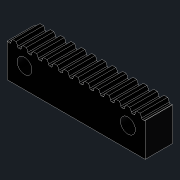
# Autodesk Inventor part: base37
Saved by Autodesk Inventor 2022 (Build 260153000, 153)
## iProperties
Created: 2021-08-06
Part Number: base37
Material: ABS プラスチック
Document SubType Name: Modeling
Designer: yuta0
Density: 1.06 g/cm^3
Appearance: 滑らか - 黒
Mass: 7.28168 g
Surface Area: 31.8793 cm^2
Volume: 6.86951 cm^3
購入先: 印刷
在庫数: 0.0
Author: yuta0
Autodesk Inventor part; units mm, degrees
(part 1 of 2)
ref_plane "YZ Plane" through (0, 0, 0) normal (1, 0, 0) x (0, 1, 0)
ref_plane "XZ Plane" through (0, 0, 0) normal (0, 1, 0) x (-1, 0, 0)
ref_plane "XY Plane" through (0, 0, 0) normal (0, 0, 1) x (1, 0, 0)
sketch "スケッチ1" plane through (0, 0, 0) normal (0, 0, 1) x (1, 0, 0)
  line L0 (-20, -5) -> (20, -5)
  line L1 (20, -5) -> (20, 9)
  line L2 (20, 9) -> (-20, 9)
  line L3 (-20, 9) -> (-20, -5)
  point P0 (0, 0)
  dimension "d0" = 40
  dimension "d66" = 5
  dimension "d67" = 9
  dimension "d68" = 20
  constraints: 8 end point, 2 parallel, 1 horizontal, 1 perpendicular
  measures "d0" distance of L0.start L0.end
  measures "d66" distance from line of L0 point (0, 0)
  measures "d67" distance from line of L2 point (0, 0)
  measures "d68" distance from line of L1 point (0, 0)
extrude "押し出し1" add sketch "スケッチ1" along normal blind 8
sketch "スケッチ2" plane through (0, 0, 8) normal (0, 0, 1) x (1, 0, 0)
  line L0 (-50, -10) -> (50, -10) construction
  line L1 (-50, -26.2338) -> (50, -26.2338) construction
  line L2 (50, 6.2338) -> (-50, 6.2338) construction
  arc A0 (-50, 6.2338) -> (-50, -26.2338) centre (-50, -10) ccw construction
  arc A1 (50, -26.2338) -> (50, 6.2338) centre (50, -10) ccw construction
  line L3 (-50, 6.6528) -> (50, 6.6528)
  arc A2 (50, -26.6528) -> (50, 6.6528) centre (50, -10) ccw
  line L4 (50, -26.6528) -> (-50, -26.6528)
  arc A3 (-50, 6.6528) -> (-50, -26.6528) centre (-50, -10) ccw
  line L5 (-50, -25.8528) -> (50, -25.8528)
  arc A4 (50, -25.8528) -> (50, 5.8528) centre (50, -10) ccw
  line L6 (50, 5.8528) -> (-50, 5.8528) construction
  arc A5 (-50, 5.8528) -> (-50, -25.8528) centre (-50, -10) ccw
  line L7 (-1.5, 4.6028) -> (-1.2549, 4.6028)
  arc A6 (-1.2549, 4.6028) -> (-0.9576, 4.8628) centre (-1.2549, 4.9028) ccw
  arc A7 (-0.5217, 5.8528) -> (-0.9576, 4.8628) centre (0.975, 4.6028) ccw
  line L8 (-0.5217, 5.8528) -> (0.5217, 5.8528)
  arc A8 (0.9576, 4.8628) -> (0.5217, 5.8528) centre (-0.975, 4.6028) ccw
  arc A9 (0.9576, 4.8628) -> (1.2549, 4.6028) centre (1.2549, 4.9028) ccw
  line L9 (1.2549, 4.6028) -> (1.5, 4.6028)
  line L10 (-20, 9) -> (-20, -5) projected
  line L11 (20, 9) -> (-20, 9) projected
  line L12 (20, -5) -> (20, 9) projected
  arc A10 (-2.0424, 4.8628) -> (-1.7451, 4.6028) centre (-1.7451, 4.9028) ccw
  arc A11 (-4.2549, 4.6028) -> (-3.9576, 4.8628) centre (-4.2549, 4.9028) ccw
  line L13 (-4.5, 4.6028) -> (-4.2549, 4.6028)
  line L14 (-1.7451, 4.6028) -> (-1.5, 4.6028)
  arc A12 (-2.0424, 4.8628) -> (-2.4783, 5.8528) centre (-3.975, 4.6028) ccw
  line L15 (-3.5217, 5.8528) -> (-2.4783, 5.8528)
  arc A13 (-3.5217, 5.8528) -> (-3.9576, 4.8628) centre (-2.025, 4.6028) ccw
  arc A14 (-5.0424, 4.8628) -> (-4.7451, 4.6028) centre (-4.7451, 4.9028) ccw
  arc A15 (-7.2549, 4.6028) -> (-6.9576, 4.8628) centre (-7.2549, 4.9028) ccw
  line L16 (-7.5, 4.6028) -> (-7.2549, 4.6028)
  line L17 (-4.7451, 4.6028) -> (-4.5, 4.6028)
  arc A16 (-5.0424, 4.8628) -> (-5.4783, 5.8528) centre (-6.975, 4.6028) ccw
  line L18 (-6.5217, 5.8528) -> (-5.4783, 5.8528)
  arc A17 (-6.5217, 5.8528) -> (-6.9576, 4.8628) centre (-5.025, 4.6028) ccw
  arc A18 (-8.0424, 4.8628) -> (-7.7451, 4.6028) centre (-7.7451, 4.9028) ccw
  arc A19 (-10.2549, 4.6028) -> (-9.9576, 4.8628) centre (-10.2549, 4.9028) ccw
  line L19 (-10.5, 4.6028) -> (-10.2549, 4.6028)
  line L20 (-7.7451, 4.6028) -> (-7.5, 4.6028)
  arc A20 (-8.0424, 4.8628) -> (-8.4783, 5.8528) centre (-9.975, 4.6028) ccw
  line L21 (-9.5217, 5.8528) -> (-8.4783, 5.8528)
  arc A21 (-9.5217, 5.8528) -> (-9.9576, 4.8628) centre (-8.025, 4.6028) ccw
  arc A22 (-11.0424, 4.8628) -> (-10.7451, 4.6028) centre (-10.7451, 4.9028) ccw
  arc A23 (-13.2549, 4.6028) -> (-12.9576, 4.8628) centre (-13.2549, 4.9028) ccw
  line L22 (-13.5, 4.6028) -> (-13.2549, 4.6028)
  line L23 (-10.7451, 4.6028) -> (-10.5, 4.6028)
  arc A24 (-11.0424, 4.8628) -> (-11.4783, 5.8528) centre (-12.975, 4.6028) ccw
  line L24 (-12.5217, 5.8528) -> (-11.4783, 5.8528)
  arc A25 (-12.5217, 5.8528) -> (-12.9576, 4.8628) centre (-11.025, 4.6028) ccw
  arc A26 (-14.0424, 4.8628) -> (-13.7451, 4.6028) centre (-13.7451, 4.9028) ccw
  arc A27 (-16.2549, 4.6028) -> (-15.9576, 4.8628) centre (-16.2549, 4.9028) ccw
  line L25 (-16.5, 4.6028) -> (-16.2549, 4.6028)
  line L26 (-13.7451, 4.6028) -> (-13.5, 4.6028)
  arc A28 (-14.0424, 4.8628) -> (-14.4783, 5.8528) centre (-15.975, 4.6028) ccw
  line L27 (-15.5217, 5.8528) -> (-14.4783, 5.8528)
  arc A29 (-15.5217, 5.8528) -> (-15.9576, 4.8628) centre (-14.025, 4.6028) ccw
  arc A30 (-17.0424, 4.8628) -> (-16.7451, 4.6028) centre (-16.7451, 4.9028) ccw
  arc A31 (-19.2549, 4.6028) -> (-18.9576, 4.8628) centre (-19.2549, 4.9028) ccw
  line L28 (-19.5, 4.6028) -> (-19.2549, 4.6028)
  line L29 (-16.7451, 4.6028) -> (-16.5, 4.6028)
  arc A32 (-17.0424, 4.8628) -> (-17.4783, 5.8528) centre (-18.975, 4.6028) ccw
  line L30 (-18.5217, 5.8528) -> (-17.4783, 5.8528)
  arc A33 (-18.5217, 5.8528) -> (-18.9576, 4.8628) centre (-17.025, 4.6028) ccw
  arc A34 (-20.0424, 4.8628) -> (-19.7451, 4.6028) centre (-19.7451, 4.9028) ccw
  arc A35 (-22.2549, 4.6028) -> (-21.9576, 4.8628) centre (-22.2549, 4.9028) ccw
  line L31 (-22.5, 4.6028) -> (-22.2549, 4.6028)
  line L32 (-19.7451, 4.6028) -> (-19.5, 4.6028)
  arc A36 (-20.0424, 4.8628) -> (-20.4783, 5.8528) centre (-21.975, 4.6028) ccw
  line L33 (-21.5217, 5.8528) -> (-20.4783, 5.8528)
  arc A37 (-21.5217, 5.8528) -> (-21.9576, 4.8628) centre (-20.025, 4.6028) ccw
  arc A38 (-23.0424, 4.8628) -> (-22.7451, 4.6028) centre (-22.7451, 4.9028) ccw
  arc A39 (-25.2549, 4.6028) -> (-24.9576, 4.8628) centre (-25.2549, 4.9028) ccw
  line L34 (-25.5, 4.6028) -> (-25.2549, 4.6028)
  line L35 (-22.7451, 4.6028) -> (-22.5, 4.6028)
  arc A40 (-23.0424, 4.8628) -> (-23.4783, 5.8528) centre (-24.975, 4.6028) ccw
  line L36 (-24.5217, 5.8528) -> (-23.4783, 5.8528)
  arc A41 (-24.5217, 5.8528) -> (-24.9576, 4.8628) centre (-23.025, 4.6028) ccw
  arc A42 (-26.0424, 4.8628) -> (-25.7451, 4.6028) centre (-25.7451, 4.9028) ccw
  arc A43 (-28.2549, 4.6028) -> (-27.9576, 4.8628) centre (-28.2549, 4.9028) ccw
  line L37 (-28.5, 4.6028) -> (-28.2549, 4.6028)
  line L38 (-25.7451, 4.6028) -> (-25.5, 4.6028)
  arc A44 (-26.0424, 4.8628) -> (-26.4783, 5.8528) centre (-27.975, 4.6028) ccw
  line L39 (-27.5217, 5.8528) -> (-26.4783, 5.8528)
  arc A45 (-27.5217, 5.8528) -> (-27.9576, 4.8628) centre (-26.025, 4.6028) ccw
  arc A46 (3.9576, 4.8628) -> (4.2549, 4.6028) centre (4.2549, 4.9028) ccw
  arc A47 (1.7451, 4.6028) -> (2.0424, 4.8628) centre (1.7451, 4.9028) ccw
  line L40 (1.5, 4.6028) -> (1.7451, 4.6028)
  line L41 (4.2549, 4.6028) -> (4.5, 4.6028)
  arc A48 (3.9576, 4.8628) -> (3.5217, 5.8528) centre (2.025, 4.6028) ccw
  line L42 (2.4783, 5.8528) -> (3.5217, 5.8528)
  arc A49 (2.4783, 5.8528) -> (2.0424, 4.8628) centre (3.975, 4.6028) ccw
  arc A50 (0.9576, 4.8628) -> (1.2549, 4.6028) centre (1.2549, 4.9028) ccw
  arc A51 (-1.2549, 4.6028) -> (-0.9576, 4.8628) centre (-1.2549, 4.9028) ccw
  line L43 (-1.5, 4.6028) -> (-1.2549, 4.6028)
  line L44 (1.2549, 4.6028) -> (1.5, 4.6028)
  arc A52 (0.9576, 4.8628) -> (0.5217, 5.8528) centre (-0.975, 4.6028) ccw
  line L45 (-0.5217, 5.8528) -> (0.5217, 5.8528)
  arc A53 (-0.5217, 5.8528) -> (-0.9576, 4.8628) centre (0.975, 4.6028) ccw
  arc A54 (-2.0424, 4.8628) -> (-1.7451, 4.6028) centre (-1.7451, 4.9028) ccw
  arc A55 (-4.2549, 4.6028) -> (-3.9576, 4.8628) centre (-4.2549, 4.9028) ccw
  line L46 (-4.5, 4.6028) -> (-4.2549, 4.6028)
  line L47 (-1.7451, 4.6028) -> (-1.5, 4.6028)
  arc A56 (-2.0424, 4.8628) -> (-2.4783, 5.8528) centre (-3.975, 4.6028) ccw
  line L48 (-3.5217, 5.8528) -> (-2.4783, 5.8528)
  arc A57 (-3.5217, 5.8528) -> (-3.9576, 4.8628) centre (-2.025, 4.6028) ccw
  arc A58 (-5.0424, 4.8628) -> (-4.7451, 4.6028) centre (-4.7451, 4.9028) ccw
  arc A59 (-7.2549, 4.6028) -> (-6.9576, 4.8628) centre (-7.2549, 4.9028) ccw
  line L49 (-7.5, 4.6028) -> (-7.2549, 4.6028)
  line L50 (-4.7451, 4.6028) -> (-4.5, 4.6028)
  arc A60 (-5.0424, 4.8628) -> (-5.4783, 5.8528) centre (-6.975, 4.6028) ccw
  line L51 (-6.5217, 5.8528) -> (-5.4783, 5.8528)
  arc A61 (-6.5217, 5.8528) -> (-6.9576, 4.8628) centre (-5.025, 4.6028) ccw
  arc A62 (-8.0424, 4.8628) -> (-7.7451, 4.6028) centre (-7.7451, 4.9028) ccw
  arc A63 (-10.2549, 4.6028) -> (-9.9576, 4.8628) centre (-10.2549, 4.9028) ccw
  line L52 (-10.5, 4.6028) -> (-10.2549, 4.6028)
  line L53 (-7.7451, 4.6028) -> (-7.5, 4.6028)
  arc A64 (-8.0424, 4.8628) -> (-8.4783, 5.8528) centre (-9.975, 4.6028) ccw
  line L54 (-9.5217, 5.8528) -> (-8.4783, 5.8528)
  arc A65 (-9.5217, 5.8528) -> (-9.9576, 4.8628) centre (-8.025, 4.6028) ccw
  arc A66 (-11.0424, 4.8628) -> (-10.7451, 4.6028) centre (-10.7451, 4.9028) ccw
  arc A67 (-13.2549, 4.6028) -> (-12.9576, 4.8628) centre (-13.2549, 4.9028) ccw
  line L55 (-13.5, 4.6028) -> (-13.2549, 4.6028)
  line L56 (-10.7451, 4.6028) -> (-10.5, 4.6028)
  arc A68 (-11.0424, 4.8628) -> (-11.4783, 5.8528) centre (-12.975, 4.6028) ccw
  line L57 (-12.5217, 5.8528) -> (-11.4783, 5.8528)
  arc A69 (-12.5217, 5.8528) -> (-12.9576, 4.8628) centre (-11.025, 4.6028) ccw
  arc A70 (-14.0424, 4.8628) -> (-13.7451, 4.6028) centre (-13.7451, 4.9028) ccw
  arc A71 (-16.2549, 4.6028) -> (-15.9576, 4.8628) centre (-16.2549, 4.9028) ccw
  line L58 (-16.5, 4.6028) -> (-16.2549, 4.6028)
  line L59 (-13.7451, 4.6028) -> (-13.5, 4.6028)
  arc A72 (-14.0424, 4.8628) -> (-14.4783, 5.8528) centre (-15.975, 4.6028) ccw
  line L60 (-15.5217, 5.8528) -> (-14.4783, 5.8528)
  arc A73 (-15.5217, 5.8528) -> (-15.9576, 4.8628) centre (-14.025, 4.6028) ccw
  arc A74 (-17.0424, 4.8628) -> (-16.7451, 4.6028) centre (-16.7451, 4.9028) ccw
  arc A75 (-19.2549, 4.6028) -> (-18.9576, 4.8628) centre (-19.2549, 4.9028) ccw
  line L61 (-19.5, 4.6028) -> (-19.2549, 4.6028)
  line L62 (-16.7451, 4.6028) -> (-16.5, 4.6028)
  arc A76 (-17.0424, 4.8628) -> (-17.4783, 5.8528) centre (-18.975, 4.6028) ccw
  line L63 (-18.5217, 5.8528) -> (-17.4783, 5.8528)
  arc A77 (-18.5217, 5.8528) -> (-18.9576, 4.8628) centre (-17.025, 4.6028) ccw
  arc A78 (-20.0424, 4.8628) -> (-19.7451, 4.6028) centre (-19.7451, 4.9028) ccw
  arc A79 (-22.2549, 4.6028) -> (-21.9576, 4.8628) centre (-22.2549, 4.9028) ccw
  line L64 (-22.5, 4.6028) -> (-22.2549, 4.6028)
  line L65 (-19.7451, 4.6028) -> (-19.5, 4.6028)
  arc A80 (-20.0424, 4.8628) -> (-20.4783, 5.8528) centre (-21.975, 4.6028) ccw
  line L66 (-21.5217, 5.8528) -> (-20.4783, 5.8528)
  arc A81 (-21.5217, 5.8528) -> (-21.9576, 4.8628) centre (-20.025, 4.6028) ccw
  arc A82 (-23.0424, 4.8628) -> (-22.7451, 4.6028) centre (-22.7451, 4.9028) ccw
  arc A83 (-25.2549, 4.6028) -> (-24.9576, 4.8628) centre (-25.2549, 4.9028) ccw
  line L67 (-25.5, 4.6028) -> (-25.2549, 4.6028)
  line L68 (-22.7451, 4.6028) -> (-22.5, 4.6028)
  arc A84 (-23.0424, 4.8628) -> (-23.4783, 5.8528) centre (-24.975, 4.6028) ccw
  line L69 (-24.5217, 5.8528) -> (-23.4783, 5.8528)
  arc A85 (-24.5217, 5.8528) -> (-24.9576, 4.8628) centre (-23.025, 4.6028) ccw
  arc A86 (6.9576, 4.8628) -> (7.2549, 4.6028) centre (7.2549, 4.9028) ccw
  arc A87 (4.7451, 4.6028) -> (5.0424, 4.8628) centre (4.7451, 4.9028) ccw
  line L70 (4.5, 4.6028) -> (4.7451, 4.6028)
  line L71 (7.2549, 4.6028) -> (7.5, 4.6028)
  arc A88 (6.9576, 4.8628) -> (6.5217, 5.8528) centre (5.025, 4.6028) ccw
  line L72 (5.4783, 5.8528) -> (6.5217, 5.8528)
  arc A89 (5.4783, 5.8528) -> (5.0424, 4.8628) centre (6.975, 4.6028) ccw
  arc A90 (3.9576, 4.8628) -> (4.2549, 4.6028) centre (4.2549, 4.9028) ccw
  arc A91 (1.7451, 4.6028) -> (2.0424, 4.8628) centre (1.7451, 4.9028) ccw
  line L73 (1.5, 4.6028) -> (1.7451, 4.6028)
  line L74 (4.2549, 4.6028) -> (4.5, 4.6028)
  arc A92 (3.9576, 4.8628) -> (3.5217, 5.8528) centre (2.025, 4.6028) ccw
  line L75 (2.4783, 5.8528) -> (3.5217, 5.8528)
  arc A93 (2.4783, 5.8528) -> (2.0424, 4.8628) centre (3.975, 4.6028) ccw
  arc A94 (0.9576, 4.8628) -> (1.2549, 4.6028) centre (1.2549, 4.9028) ccw
  arc A95 (-1.2549, 4.6028) -> (-0.9576, 4.8628) centre (-1.2549, 4.9028) ccw
  line L76 (-1.5, 4.6028) -> (-1.2549, 4.6028)
  line L77 (1.2549, 4.6028) -> (1.5, 4.6028)
  arc A96 (0.9576, 4.8628) -> (0.5217, 5.8528) centre (-0.975, 4.6028) ccw
  line L78 (-0.5217, 5.8528) -> (0.5217, 5.8528)
  arc A97 (-0.5217, 5.8528) -> (-0.9576, 4.8628) centre (0.975, 4.6028) ccw
  arc A98 (-2.0424, 4.8628) -> (-1.7451, 4.6028) centre (-1.7451, 4.9028) ccw
  arc A99 (-4.2549, 4.6028) -> (-3.9576, 4.8628) centre (-4.2549, 4.9028) ccw
  line L79 (-4.5, 4.6028) -> (-4.2549, 4.6028)
  line L80 (-1.7451, 4.6028) -> (-1.5, 4.6028)
  arc A100 (-2.0424, 4.8628) -> (-2.4783, 5.8528) centre (-3.975, 4.6028) ccw
  line L81 (-3.5217, 5.8528) -> (-2.4783, 5.8528)
  arc A101 (-3.5217, 5.8528) -> (-3.9576, 4.8628) centre (-2.025, 4.6028) ccw
  arc A102 (-5.0424, 4.8628) -> (-4.7451, 4.6028) centre (-4.7451, 4.9028) ccw
  arc A103 (-7.2549, 4.6028) -> (-6.9576, 4.8628) centre (-7.2549, 4.9028) ccw
  line L82 (-7.5, 4.6028) -> (-7.2549, 4.6028)
  line L83 (-4.7451, 4.6028) -> (-4.5, 4.6028)
  arc A104 (-5.0424, 4.8628) -> (-5.4783, 5.8528) centre (-6.975, 4.6028) ccw
  line L84 (-6.5217, 5.8528) -> (-5.4783, 5.8528)
  arc A105 (-6.5217, 5.8528) -> (-6.9576, 4.8628) centre (-5.025, 4.6028) ccw
  arc A106 (-8.0424, 4.8628) -> (-7.7451, 4.6028) centre (-7.7451, 4.9028) ccw
  arc A107 (-10.2549, 4.6028) -> (-9.9576, 4.8628) centre (-10.2549, 4.9028) ccw
  line L85 (-10.5, 4.6028) -> (-10.2549, 4.6028)
  line L86 (-7.7451, 4.6028) -> (-7.5, 4.6028)
  arc A108 (-8.0424, 4.8628) -> (-8.4783, 5.8528) centre (-9.975, 4.6028) ccw
  line L87 (-9.5217, 5.8528) -> (-8.4783, 5.8528)
  arc A109 (-9.5217, 5.8528) -> (-9.9576, 4.8628) centre (-8.025, 4.6028) ccw
  arc A110 (-11.0424, 4.8628) -> (-10.7451, 4.6028) centre (-10.7451, 4.9028) ccw
  arc A111 (-13.2549, 4.6028) -> (-12.9576, 4.8628) centre (-13.2549, 4.9028) ccw
  line L88 (-13.5, 4.6028) -> (-13.2549, 4.6028)
  line L89 (-10.7451, 4.6028) -> (-10.5, 4.6028)
  arc A112 (-11.0424, 4.8628) -> (-11.4783, 5.8528) centre (-12.975, 4.6028) ccw
  line L90 (-12.5217, 5.8528) -> (-11.4783, 5.8528)
  arc A113 (-12.5217, 5.8528) -> (-12.9576, 4.8628) centre (-11.025, 4.6028) ccw
  arc A114 (-14.0424, 4.8628) -> (-13.7451, 4.6028) centre (-13.7451, 4.9028) ccw
  arc A115 (-16.2549, 4.6028) -> (-15.9576, 4.8628) centre (-16.2549, 4.9028) ccw
  line L91 (-16.5, 4.6028) -> (-16.2549, 4.6028)
  line L92 (-13.7451, 4.6028) -> (-13.5, 4.6028)
  arc A116 (-14.0424, 4.8628) -> (-14.4783, 5.8528) centre (-15.975, 4.6028) ccw
  line L93 (-15.5217, 5.8528) -> (-14.4783, 5.8528)
  arc A117 (-15.5217, 5.8528) -> (-15.9576, 4.8628) centre (-14.025, 4.6028) ccw
  arc A118 (-17.0424, 4.8628) -> (-16.7451, 4.6028) centre (-16.7451, 4.9028) ccw
  arc A119 (-19.2549, 4.6028) -> (-18.9576, 4.8628) centre (-19.2549, 4.9028) ccw
  line L94 (-19.5, 4.6028) -> (-19.2549, 4.6028)
  line L95 (-16.7451, 4.6028) -> (-16.5, 4.6028)
  arc A120 (-17.0424, 4.8628) -> (-17.4783, 5.8528) centre (-18.975, 4.6028) ccw
  line L96 (-18.5217, 5.8528) -> (-17.4783, 5.8528)
  arc A121 (-18.5217, 5.8528) -> (-18.9576, 4.8628) centre (-17.025, 4.6028) ccw
  arc A122 (-20.0424, 4.8628) -> (-19.7451, 4.6028) centre (-19.7451, 4.9028) ccw
  arc A123 (-22.2549, 4.6028) -> (-21.9576, 4.8628) centre (-22.2549, 4.9028) ccw
  line L97 (-22.5, 4.6028) -> (-22.2549, 4.6028)
  line L98 (-19.7451, 4.6028) -> (-19.5, 4.6028)
  arc A124 (-20.0424, 4.8628) -> (-20.4783, 5.8528) centre (-21.975, 4.6028) ccw
  line L99 (-21.5217, 5.8528) -> (-20.4783, 5.8528)
  arc A125 (-21.5217, 5.8528) -> (-21.9576, 4.8628) centre (-20.025, 4.6028) ccw
  arc A126 (9.9576, 4.8628) -> (10.2549, 4.6028) centre (10.2549, 4.9028) ccw
  arc A127 (7.7451, 4.6028) -> (8.0424, 4.8628) centre (7.7451, 4.9028) ccw
  line L100 (7.5, 4.6028) -> (7.7451, 4.6028)
  line L101 (10.2549, 4.6028) -> (10.5, 4.6028)
  arc A128 (9.9576, 4.8628) -> (9.5217, 5.8528) centre (8.025, 4.6028) ccw
  line L102 (8.4783, 5.8528) -> (9.5217, 5.8528)
  arc A129 (8.4783, 5.8528) -> (8.0424, 4.8628) centre (9.975, 4.6028) ccw
  arc A130 (6.9576, 4.8628) -> (7.2549, 4.6028) centre (7.2549, 4.9028) ccw
  arc A131 (4.7451, 4.6028) -> (5.0424, 4.8628) centre (4.7451, 4.9028) ccw
  line L103 (4.5, 4.6028) -> (4.7451, 4.6028)
  line L104 (7.2549, 4.6028) -> (7.5, 4.6028)
  arc A132 (6.9576, 4.8628) -> (6.5217, 5.8528) centre (5.025, 4.6028) ccw
  line L105 (5.4783, 5.8528) -> (6.5217, 5.8528)
  arc A133 (5.4783, 5.8528) -> (5.0424, 4.8628) centre (6.975, 4.6028) ccw
  arc A134 (3.9576, 4.8628) -> (4.2549, 4.6028) centre (4.2549, 4.9028) ccw
  arc A135 (1.7451, 4.6028) -> (2.0424, 4.8628) centre (1.7451, 4.9028) ccw
  line L106 (1.5, 4.6028) -> (1.7451, 4.6028)
  line L107 (4.2549, 4.6028) -> (4.5, 4.6028)
  arc A136 (3.9576, 4.8628) -> (3.5217, 5.8528) centre (2.025, 4.6028) ccw
  line L108 (2.4783, 5.8528) -> (3.5217, 5.8528)
  arc A137 (2.4783, 5.8528) -> (2.0424, 4.8628) centre (3.975, 4.6028) ccw
  arc A138 (0.9576, 4.8628) -> (1.2549, 4.6028) centre (1.2549, 4.9028) ccw
  arc A139 (-1.2549, 4.6028) -> (-0.9576, 4.8628) centre (-1.2549, 4.9028) ccw
  line L109 (-1.5, 4.6028) -> (-1.2549, 4.6028)
  line L110 (1.2549, 4.6028) -> (1.5, 4.6028)
  arc A140 (0.9576, 4.8628) -> (0.5217, 5.8528) centre (-0.975, 4.6028) ccw
  line L111 (-0.5217, 5.8528) -> (0.5217, 5.8528)
  arc A141 (-0.5217, 5.8528) -> (-0.9576, 4.8628) centre (0.975, 4.6028) ccw
  arc A142 (-2.0424, 4.8628) -> (-1.7451, 4.6028) centre (-1.7451, 4.9028) ccw
  arc A143 (-4.2549, 4.6028) -> (-3.9576, 4.8628) centre (-4.2549, 4.9028) ccw
  line L112 (-4.5, 4.6028) -> (-4.2549, 4.6028)
  line L113 (-1.7451, 4.6028) -> (-1.5, 4.6028)
  arc A144 (-2.0424, 4.8628) -> (-2.4783, 5.8528) centre (-3.975, 4.6028) ccw
  line L114 (-3.5217, 5.8528) -> (-2.4783, 5.8528)
  arc A145 (-3.5217, 5.8528) -> (-3.9576, 4.8628) centre (-2.025, 4.6028) ccw
  arc A146 (-5.0424, 4.8628) -> (-4.7451, 4.6028) centre (-4.7451, 4.9028) ccw
  arc A147 (-7.2549, 4.6028) -> (-6.9576, 4.8628) centre (-7.2549, 4.9028) ccw
  line L115 (-7.5, 4.6028) -> (-7.2549, 4.6028)
  line L116 (-4.7451, 4.6028) -> (-4.5, 4.6028)
  arc A148 (-5.0424, 4.8628) -> (-5.4783, 5.8528) centre (-6.975, 4.6028) ccw
  line L117 (-6.5217, 5.8528) -> (-5.4783, 5.8528)
  arc A149 (-6.5217, 5.8528) -> (-6.9576, 4.8628) centre (-5.025, 4.6028) ccw
  arc A150 (-8.0424, 4.8628) -> (-7.7451, 4.6028) centre (-7.7451, 4.9028) ccw
  arc A151 (-10.2549, 4.6028) -> (-9.9576, 4.8628) centre (-10.2549, 4.9028) ccw
  line L118 (-10.5, 4.6028) -> (-10.2549, 4.6028)
  line L119 (-7.7451, 4.6028) -> (-7.5, 4.6028)
  arc A152 (-8.0424, 4.8628) -> (-8.4783, 5.8528) centre (-9.975, 4.6028) ccw
  line L120 (-9.5217, 5.8528) -> (-8.4783, 5.8528)
  arc A153 (-9.5217, 5.8528) -> (-9.9576, 4.8628) centre (-8.025, 4.6028) ccw
  arc A154 (-11.0424, 4.8628) -> (-10.7451, 4.6028) centre (-10.7451, 4.9028) ccw
  arc A155 (-13.2549, 4.6028) -> (-12.9576, 4.8628) centre (-13.2549, 4.9028) ccw
  line L121 (-13.5, 4.6028) -> (-13.2549, 4.6028)
  line L122 (-10.7451, 4.6028) -> (-10.5, 4.6028)
  arc A156 (-11.0424, 4.8628) -> (-11.4783, 5.8528) centre (-12.975, 4.6028) ccw
  line L123 (-12.5217, 5.8528) -> (-11.4783, 5.8528)
  arc A157 (-12.5217, 5.8528) -> (-12.9576, 4.8628) centre (-11.025, 4.6028) ccw
  arc A158 (-14.0424, 4.8628) -> (-13.7451, 4.6028) centre (-13.7451, 4.9028) ccw
  arc A159 (-16.2549, 4.6028) -> (-15.9576, 4.8628) centre (-16.2549, 4.9028) ccw
  line L124 (-16.5, 4.6028) -> (-16.2549, 4.6028)
  line L125 (-13.7451, 4.6028) -> (-13.5, 4.6028)
  arc A160 (-14.0424, 4.8628) -> (-14.4783, 5.8528) centre (-15.975, 4.6028) ccw
  line L126 (-15.5217, 5.8528) -> (-14.4783, 5.8528)
  arc A161 (-15.5217, 5.8528) -> (-15.9576, 4.8628) centre (-14.025, 4.6028) ccw
  arc A162 (-17.0424, 4.8628) -> (-16.7451, 4.6028) centre (-16.7451, 4.9028) ccw
  arc A163 (-19.2549, 4.6028) -> (-18.9576, 4.8628) centre (-19.2549, 4.9028) ccw
  line L127 (-19.5, 4.6028) -> (-19.2549, 4.6028)
  line L128 (-16.7451, 4.6028) -> (-16.5, 4.6028)
  arc A164 (-17.0424, 4.8628) -> (-17.4783, 5.8528) centre (-18.975, 4.6028) ccw
  line L129 (-18.5217, 5.8528) -> (-17.4783, 5.8528)
  arc A165 (-18.5217, 5.8528) -> (-18.9576, 4.8628) centre (-17.025, 4.6028) ccw
  arc A166 (12.9576, 4.8628) -> (13.2549, 4.6028) centre (13.2549, 4.9028) ccw
  arc A167 (10.7451, 4.6028) -> (11.0424, 4.8628) centre (10.7451, 4.9028) ccw
  line L130 (10.5, 4.6028) -> (10.7451, 4.6028)
  line L131 (13.2549, 4.6028) -> (13.5, 4.6028)
  arc A168 (12.9576, 4.8628) -> (12.5217, 5.8528) centre (11.025, 4.6028) ccw
  line L132 (11.4783, 5.8528) -> (12.5217, 5.8528)
  arc A169 (11.4783, 5.8528) -> (11.0424, 4.8628) centre (12.975, 4.6028) ccw
  arc A170 (9.9576, 4.8628) -> (10.2549, 4.6028) centre (10.2549, 4.9028) ccw
  arc A171 (7.7451, 4.6028) -> (8.0424, 4.8628) centre (7.7451, 4.9028) ccw
  line L133 (7.5, 4.6028) -> (7.7451, 4.6028)
  line L134 (10.2549, 4.6028) -> (10.5, 4.6028)
  arc A172 (9.9576, 4.8628) -> (9.5217, 5.8528) centre (8.025, 4.6028) ccw
  line L135 (8.4783, 5.8528) -> (9.5217, 5.8528)
  arc A173 (8.4783, 5.8528) -> (8.0424, 4.8628) centre (9.975, 4.6028) ccw
  arc A174 (6.9576, 4.8628) -> (7.2549, 4.6028) centre (7.2549, 4.9028) ccw
  arc A175 (4.7451, 4.6028) -> (5.0424, 4.8628) centre (4.7451, 4.9028) ccw
  line L136 (4.5, 4.6028) -> (4.7451, 4.6028)
  line L137 (7.2549, 4.6028) -> (7.5, 4.6028)
  arc A176 (6.9576, 4.8628) -> (6.5217, 5.8528) centre (5.025, 4.6028) ccw
  line L138 (5.4783, 5.8528) -> (6.5217, 5.8528)
  arc A177 (5.4783, 5.8528) -> (5.0424, 4.8628) centre (6.975, 4.6028) ccw
  arc A178 (3.9576, 4.8628) -> (4.2549, 4.6028) centre (4.2549, 4.9028) ccw
  arc A179 (1.7451, 4.6028) -> (2.0424, 4.8628) centre (1.7451, 4.9028) ccw
  line L139 (1.5, 4.6028) -> (1.7451, 4.6028)
  line L140 (4.2549, 4.6028) -> (4.5, 4.6028)
  arc A180 (3.9576, 4.8628) -> (3.5217, 5.8528) centre (2.025, 4.6028) ccw
  line L141 (2.4783, 5.8528) -> (3.5217, 5.8528)
  arc A181 (2.4783, 5.8528) -> (2.0424, 4.8628) centre (3.975, 4.6028) ccw
  arc A182 (0.9576, 4.8628) -> (1.2549, 4.6028) centre (1.2549, 4.9028) ccw
  arc A183 (-1.2549, 4.6028) -> (-0.9576, 4.8628) centre (-1.2549, 4.9028) ccw
  line L142 (-1.5, 4.6028) -> (-1.2549, 4.6028)
  line L143 (1.2549, 4.6028) -> (1.5, 4.6028)
  arc A184 (0.9576, 4.8628) -> (0.5217, 5.8528) centre (-0.975, 4.6028) ccw
  line L144 (-0.5217, 5.8528) -> (0.5217, 5.8528)
  arc A185 (-0.5217, 5.8528) -> (-0.9576, 4.8628) centre (0.975, 4.6028) ccw
  arc A186 (-2.0424, 4.8628) -> (-1.7451, 4.6028) centre (-1.7451, 4.9028) ccw
  arc A187 (-4.2549, 4.6028) -> (-3.9576, 4.8628) centre (-4.2549, 4.9028) ccw
  line L145 (-4.5, 4.6028) -> (-4.2549, 4.6028)
  line L146 (-1.7451, 4.6028) -> (-1.5, 4.6028)
  arc A188 (-2.0424, 4.8628) -> (-2.4783, 5.8528) centre (-3.975, 4.6028) ccw
  line L147 (-3.5217, 5.8528) -> (-2.4783, 5.8528)
  arc A189 (-3.5217, 5.8528) -> (-3.9576, 4.8628) centre (-2.025, 4.6028) ccw
  arc A190 (-5.0424, 4.8628) -> (-4.7451, 4.6028) centre (-4.7451, 4.9028) ccw
  arc A191 (-7.2549, 4.6028) -> (-6.9576, 4.8628) centre (-7.2549, 4.9028) ccw
  line L148 (-7.5, 4.6028) -> (-7.2549, 4.6028)
  line L149 (-4.7451, 4.6028) -> (-4.5, 4.6028)
  arc A192 (-5.0424, 4.8628) -> (-5.4783, 5.8528) centre (-6.975, 4.6028) ccw
  line L150 (-6.5217, 5.8528) -> (-5.4783, 5.8528)
  arc A193 (-6.5217, 5.8528) -> (-6.9576, 4.8628) centre (-5.025, 4.6028) ccw
  arc A194 (-8.0424, 4.8628) -> (-7.7451, 4.6028) centre (-7.7451, 4.9028) ccw
  arc A195 (-10.2549, 4.6028) -> (-9.9576, 4.8628) centre (-10.2549, 4.9028) ccw
  line L151 (-10.5, 4.6028) -> (-10.2549, 4.6028)
  line L152 (-7.7451, 4.6028) -> (-7.5, 4.6028)
  arc A196 (-8.0424, 4.8628) -> (-8.4783, 5.8528) centre (-9.975, 4.6028) ccw
  line L153 (-9.5217, 5.8528) -> (-8.4783, 5.8528)
  arc A197 (-9.5217, 5.8528) -> (-9.9576, 4.8628) centre (-8.025, 4.6028) ccw
  arc A198 (-11.0424, 4.8628) -> (-10.7451, 4.6028) centre (-10.7451, 4.9028) ccw
  arc A199 (-13.2549, 4.6028) -> (-12.9576, 4.8628) centre (-13.2549, 4.9028) ccw
  line L154 (-13.5, 4.6028) -> (-13.2549, 4.6028)
  line L155 (-10.7451, 4.6028) -> (-10.5, 4.6028)
  arc A200 (-11.0424, 4.8628) -> (-11.4783, 5.8528) centre (-12.975, 4.6028) ccw
  line L156 (-12.5217, 5.8528) -> (-11.4783, 5.8528)
  arc A201 (-12.5217, 5.8528) -> (-12.9576, 4.8628) centre (-11.025, 4.6028) ccw
  arc A202 (-14.0424, 4.8628) -> (-13.7451, 4.6028) centre (-13.7451, 4.9028) ccw
  arc A203 (-16.2549, 4.6028) -> (-15.9576, 4.8628) centre (-16.2549, 4.9028) ccw
  line L157 (-16.5, 4.6028) -> (-16.2549, 4.6028)
  line L158 (-13.7451, 4.6028) -> (-13.5, 4.6028)
  arc A204 (-14.0424, 4.8628) -> (-14.4783, 5.8528) centre (-15.975, 4.6028) ccw
  line L159 (-15.5217, 5.8528) -> (-14.4783, 5.8528)
  arc A205 (-15.5217, 5.8528) -> (-15.9576, 4.8628) centre (-14.025, 4.6028) ccw
  arc A206 (15.9576, 4.8628) -> (16.2549, 4.6028) centre (16.2549, 4.9028) ccw
  arc A207 (13.7451, 4.6028) -> (14.0424, 4.8628) centre (13.7451, 4.9028) ccw
  line L160 (13.5, 4.6028) -> (13.7451, 4.6028)
  line L161 (16.2549, 4.6028) -> (16.5, 4.6028)
  arc A208 (15.9576, 4.8628) -> (15.5217, 5.8528) centre (14.025, 4.6028) ccw
  line L162 (14.4783, 5.8528) -> (15.5217, 5.8528)
  arc A209 (14.4783, 5.8528) -> (14.0424, 4.8628) centre (15.975, 4.6028) ccw
  arc A210 (12.9576, 4.8628) -> (13.2549, 4.6028) centre (13.2549, 4.9028) ccw
  arc A211 (10.7451, 4.6028) -> (11.0424, 4.8628) centre (10.7451, 4.9028) ccw
  line L163 (10.5, 4.6028) -> (10.7451, 4.6028)
  line L164 (13.2549, 4.6028) -> (13.5, 4.6028)
  arc A212 (12.9576, 4.8628) -> (12.5217, 5.8528) centre (11.025, 4.6028) ccw
  line L165 (11.4783, 5.8528) -> (12.5217, 5.8528)
  arc A213 (11.4783, 5.8528) -> (11.0424, 4.8628) centre (12.975, 4.6028) ccw
  arc A214 (9.9576, 4.8628) -> (10.2549, 4.6028) centre (10.2549, 4.9028) ccw
  arc A215 (7.7451, 4.6028) -> (8.0424, 4.8628) centre (7.7451, 4.9028) ccw
  line L166 (7.5, 4.6028) -> (7.7451, 4.6028)
  line L167 (10.2549, 4.6028) -> (10.5, 4.6028)
  arc A216 (9.9576, 4.8628) -> (9.5217, 5.8528) centre (8.025, 4.6028) ccw
  line L168 (8.4783, 5.8528) -> (9.5217, 5.8528)
  arc A217 (8.4783, 5.8528) -> (8.0424, 4.8628) centre (9.975, 4.6028) ccw
  arc A218 (6.9576, 4.8628) -> (7.2549, 4.6028) centre (7.2549, 4.9028) ccw
  arc A219 (4.7451, 4.6028) -> (5.0424, 4.8628) centre (4.7451, 4.9028) ccw
  line L169 (4.5, 4.6028) -> (4.7451, 4.6028)
  line L170 (7.2549, 4.6028) -> (7.5, 4.6028)
  arc A220 (6.9576, 4.8628) -> (6.5217, 5.8528) centre (5.025, 4.6028) ccw
  line L171 (5.4783, 5.8528) -> (6.5217, 5.8528)
  arc A221 (5.4783, 5.8528) -> (5.0424, 4.8628) centre (6.975, 4.6028) ccw
  arc A222 (3.9576, 4.8628) -> (4.2549, 4.6028) centre (4.2549, 4.9028) ccw
  arc A223 (1.7451, 4.6028) -> (2.0424, 4.8628) centre (1.7451, 4.9028) ccw
  line L172 (1.5, 4.6028) -> (1.7451, 4.6028)
  line L173 (4.2549, 4.6028) -> (4.5, 4.6028)
  arc A224 (3.9576, 4.8628) -> (3.5217, 5.8528) centre (2.025, 4.6028) ccw
  line L174 (2.4783, 5.8528) -> (3.5217, 5.8528)
  arc A225 (2.4783, 5.8528) -> (2.0424, 4.8628) centre (3.975, 4.6028) ccw
  arc A226 (0.9576, 4.8628) -> (1.2549, 4.6028) centre (1.2549, 4.9028) ccw
  arc A227 (-1.2549, 4.6028) -> (-0.9576, 4.8628) centre (-1.2549, 4.9028) ccw
  line L175 (-1.5, 4.6028) -> (-1.2549, 4.6028)
  line L176 (1.2549, 4.6028) -> (1.5, 4.6028)
  arc A228 (0.9576, 4.8628) -> (0.5217, 5.8528) centre (-0.975, 4.6028) ccw
  line L177 (-0.5217, 5.8528) -> (0.5217, 5.8528)
  arc A229 (-0.5217, 5.8528) -> (-0.9576, 4.8628) centre (0.975, 4.6028) ccw
  arc A230 (-2.0424, 4.8628) -> (-1.7451, 4.6028) centre (-1.7451, 4.9028) ccw
  arc A231 (-4.2549, 4.6028) -> (-3.9576, 4.8628) centre (-4.2549, 4.9028) ccw
  line L178 (-4.5, 4.6028) -> (-4.2549, 4.6028)
  line L179 (-1.7451, 4.6028) -> (-1.5, 4.6028)
  arc A232 (-2.0424, 4.8628) -> (-2.4783, 5.8528) centre (-3.975, 4.6028) ccw
  line L180 (-3.5217, 5.8528) -> (-2.4783, 5.8528)
  arc A233 (-3.5217, 5.8528) -> (-3.9576, 4.8628) centre (-2.025, 4.6028) ccw
  arc A234 (-5.0424, 4.8628) -> (-4.7451, 4.6028) centre (-4.7451, 4.9028) ccw
  arc A235 (-7.2549, 4.6028) -> (-6.9576, 4.8628) centre (-7.2549, 4.9028) ccw
  line L181 (-7.5, 4.6028) -> (-7.2549, 4.6028)
  line L182 (-4.7451, 4.6028) -> (-4.5, 4.6028)
  arc A236 (-5.0424, 4.8628) -> (-5.4783, 5.8528) centre (-6.975, 4.6028) ccw
  line L183 (-6.5217, 5.8528) -> (-5.4783, 5.8528)
  arc A237 (-6.5217, 5.8528) -> (-6.9576, 4.8628) centre (-5.025, 4.6028) ccw
  arc A238 (-8.0424, 4.8628) -> (-7.7451, 4.6028) centre (-7.7451, 4.9028) ccw
  arc A239 (-10.2549, 4.6028) -> (-9.9576, 4.8628) centre (-10.2549, 4.9028) ccw
  line L184 (-10.5, 4.6028) -> (-10.2549, 4.6028)
  line L185 (-7.7451, 4.6028) -> (-7.5, 4.6028)
  arc A240 (-8.0424, 4.8628) -> (-8.4783, 5.8528) centre (-9.975, 4.6028) ccw
  line L186 (-9.5217, 5.8528) -> (-8.4783, 5.8528)
  arc A241 (-9.5217, 5.8528) -> (-9.9576, 4.8628) centre (-8.025, 4.6028) ccw
  arc A242 (-11.0424, 4.8628) -> (-10.7451, 4.6028) centre (-10.7451, 4.9028) ccw
  arc A243 (-13.2549, 4.6028) -> (-12.9576, 4.8628) centre (-13.2549, 4.9028) ccw
  line L187 (-13.5, 4.6028) -> (-13.2549, 4.6028)
  line L188 (-10.7451, 4.6028) -> (-10.5, 4.6028)
  arc A244 (-11.0424, 4.8628) -> (-11.4783, 5.8528) centre (-12.975, 4.6028) ccw
  line L189 (-12.5217, 5.8528) -> (-11.4783, 5.8528)
  arc A245 (-12.5217, 5.8528) -> (-12.9576, 4.8628) centre (-11.025, 4.6028) ccw
  arc A246 (18.9576, 4.8628) -> (19.2549, 4.6028) centre (19.2549, 4.9028) ccw
  arc A247 (16.7451, 4.6028) -> (17.0424, 4.8628) centre (16.7451, 4.9028) ccw
  line L190 (16.5, 4.6028) -> (16.7451, 4.6028)
  line L191 (19.2549, 4.6028) -> (19.5, 4.6028)
  arc A248 (18.9576, 4.8628) -> (18.5217, 5.8528) centre (17.025, 4.6028) ccw
  line L192 (17.4783, 5.8528) -> (18.5217, 5.8528)
  arc A249 (17.4783, 5.8528) -> (17.0424, 4.8628) centre (18.975, 4.6028) ccw
  arc A250 (15.9576, 4.8628) -> (16.2549, 4.6028) centre (16.2549, 4.9028) ccw
  arc A251 (13.7451, 4.6028) -> (14.0424, 4.8628) centre (13.7451, 4.9028) ccw
  line L193 (13.5, 4.6028) -> (13.7451, 4.6028)
  line L194 (16.2549, 4.6028) -> (16.5, 4.6028)
  arc A252 (15.9576, 4.8628) -> (15.5217, 5.8528) centre (14.025, 4.6028) ccw
  line L195 (14.4783, 5.8528) -> (15.5217, 5.8528)
  arc A253 (14.4783, 5.8528) -> (14.0424, 4.8628) centre (15.975, 4.6028) ccw
  arc A254 (12.9576, 4.8628) -> (13.2549, 4.6028) centre (13.2549, 4.9028) ccw
  arc A255 (10.7451, 4.6028) -> (11.0424, 4.8628) centre (10.7451, 4.9028) ccw
  line L196 (10.5, 4.6028) -> (10.7451, 4.6028)
  line L197 (13.2549, 4.6028) -> (13.5, 4.6028)
  arc A256 (12.9576, 4.8628) -> (12.5217, 5.8528) centre (11.025, 4.6028) ccw
  line L198 (11.4783, 5.8528) -> (12.5217, 5.8528)
  arc A257 (11.4783, 5.8528) -> (11.0424, 4.8628) centre (12.975, 4.6028) ccw
  arc A258 (9.9576, 4.8628) -> (10.2549, 4.6028) centre (10.2549, 4.9028) ccw
  arc A259 (7.7451, 4.6028) -> (8.0424, 4.8628) centre (7.7451, 4.9028) ccw
  line L199 (7.5, 4.6028) -> (7.7451, 4.6028)
  line L200 (10.2549, 4.6028) -> (10.5, 4.6028)
  arc A260 (9.9576, 4.8628) -> (9.5217, 5.8528) centre (8.025, 4.6028) ccw
  line L201 (8.4783, 5.8528) -> (9.5217, 5.8528)
  arc A261 (8.4783, 5.8528) -> (8.0424, 4.8628) centre (9.975, 4.6028) ccw
  arc A262 (6.9576, 4.8628) -> (7.2549, 4.6028) centre (7.2549, 4.9028) ccw
  arc A263 (4.7451, 4.6028) -> (5.0424, 4.8628) centre (4.7451, 4.9028) ccw
  line L202 (4.5, 4.6028) -> (4.7451, 4.6028)
  line L203 (7.2549, 4.6028) -> (7.5, 4.6028)
  arc A264 (6.9576, 4.8628) -> (6.5217, 5.8528) centre (5.025, 4.6028) ccw
  line L204 (5.4783, 5.8528) -> (6.5217, 5.8528)
  arc A265 (5.4783, 5.8528) -> (5.0424, 4.8628) centre (6.975, 4.6028) ccw
  arc A266 (3.9576, 4.8628) -> (4.2549, 4.6028) centre (4.2549, 4.9028) ccw
  arc A267 (1.7451, 4.6028) -> (2.0424, 4.8628) centre (1.7451, 4.9028) ccw
  line L205 (1.5, 4.6028) -> (1.7451, 4.6028)
  line L206 (4.2549, 4.6028) -> (4.5, 4.6028)
  arc A268 (3.9576, 4.8628) -> (3.5217, 5.8528) centre (2.025, 4.6028) ccw
  line L207 (2.4783, 5.8528) -> (3.5217, 5.8528)
  arc A269 (2.4783, 5.8528) -> (2.0424, 4.8628) centre (3.975, 4.6028) ccw
  arc A270 (0.9576, 4.8628) -> (1.2549, 4.6028) centre (1.2549, 4.9028) ccw
  arc A271 (-1.2549, 4.6028) -> (-0.9576, 4.8628) centre (-1.2549, 4.9028) ccw
  line L208 (-1.5, 4.6028) -> (-1.2549, 4.6028)
  line L209 (1.2549, 4.6028) -> (1.5, 4.6028)
  arc A272 (0.9576, 4.8628) -> (0.5217, 5.8528) centre (-0.975, 4.6028) ccw
  line L210 (-0.5217, 5.8528) -> (0.5217, 5.8528)
  arc A273 (-0.5217, 5.8528) -> (-0.9576, 4.8628) centre (0.975, 4.6028) ccw
  arc A274 (-2.0424, 4.8628) -> (-1.7451, 4.6028) centre (-1.7451, 4.9028) ccw
  arc A275 (-4.2549, 4.6028) -> (-3.9576, 4.8628) centre (-4.2549, 4.9028) ccw
  line L211 (-4.5, 4.6028) -> (-4.2549, 4.6028)
  line L212 (-1.7451, 4.6028) -> (-1.5, 4.6028)
  arc A276 (-2.0424, 4.8628) -> (-2.4783, 5.8528) centre (-3.975, 4.6028) ccw
  line L213 (-3.5217, 5.8528) -> (-2.4783, 5.8528)
  arc A277 (-3.5217, 5.8528) -> (-3.9576, 4.8628) centre (-2.025, 4.6028) ccw
  arc A278 (-5.0424, 4.8628) -> (-4.7451, 4.6028) centre (-4.7451, 4.9028) ccw
  arc A279 (-7.2549, 4.6028) -> (-6.9576, 4.8628) centre (-7.2549, 4.9028) ccw
  line L214 (-7.5, 4.6028) -> (-7.2549, 4.6028)
  line L215 (-4.7451, 4.6028) -> (-4.5, 4.6028)
  arc A280 (-5.0424, 4.8628) -> (-5.4783, 5.8528) centre (-6.975, 4.6028) ccw
  line L216 (-6.5217, 5.8528) -> (-5.4783, 5.8528)
  arc A281 (-6.5217, 5.8528) -> (-6.9576, 4.8628) centre (-5.025, 4.6028) ccw
  arc A282 (-8.0424, 4.8628) -> (-7.7451, 4.6028) centre (-7.7451, 4.9028) ccw
  arc A283 (-10.2549, 4.6028) -> (-9.9576, 4.8628) centre (-10.2549, 4.9028) ccw
  line L217 (-10.5, 4.6028) -> (-10.2549, 4.6028)
  line L218 (-7.7451, 4.6028) -> (-7.5, 4.6028)
  arc A284 (-8.0424, 4.8628) -> (-8.4783, 5.8528) centre (-9.975, 4.6028) ccw
  line L219 (-9.5217, 5.8528) -> (-8.4783, 5.8528)
  arc A285 (-9.5217, 5.8528) -> (-9.9576, 4.8628) centre (-8.025, 4.6028) ccw
  arc A286 (21.9576, 4.8628) -> (22.2549, 4.6028) centre (22.2549, 4.9028) ccw
  arc A287 (19.7451, 4.6028) -> (20.0424, 4.8628) centre (19.7451, 4.9028) ccw
  line L220 (19.5, 4.6028) -> (19.7451, 4.6028)
  line L221 (22.2549, 4.6028) -> (22.5, 4.6028)
  arc A288 (21.9576, 4.8628) -> (21.5217, 5.8528) centre (20.025, 4.6028) ccw
  line L222 (20.4783, 5.8528) -> (21.5217, 5.8528)
  arc A289 (20.4783, 5.8528) -> (20.0424, 4.8628) centre (21.975, 4.6028) ccw
  arc A290 (18.9576, 4.8628) -> (19.2549, 4.6028) centre (19.2549, 4.9028) ccw
  arc A291 (16.7451, 4.6028) -> (17.0424, 4.8628) centre (16.7451, 4.9028) ccw
  line L223 (16.5, 4.6028) -> (16.7451, 4.6028)
  line L224 (19.2549, 4.6028) -> (19.5, 4.6028)
  arc A292 (18.9576, 4.8628) -> (18.5217, 5.8528) centre (17.025, 4.6028) ccw
  line L225 (17.4783, 5.8528) -> (18.5217, 5.8528)
  arc A293 (17.4783, 5.8528) -> (17.0424, 4.8628) centre (18.975, 4.6028) ccw
  arc A294 (15.9576, 4.8628) -> (16.2549, 4.6028) centre (16.2549, 4.9028) ccw
  arc A295 (13.7451, 4.6028) -> (14.0424, 4.8628) centre (13.7451, 4.9028) ccw
  line L226 (13.5, 4.6028) -> (13.7451, 4.6028)
  line L227 (16.2549, 4.6028) -> (16.5, 4.6028)
  arc A296 (15.9576, 4.8628) -> (15.5217, 5.8528) centre (14.025, 4.6028) ccw
  line L228 (14.4783, 5.8528) -> (15.5217, 5.8528)
  arc A297 (14.4783, 5.8528) -> (14.0424, 4.8628) centre (15.975, 4.6028) ccw
  arc A298 (12.9576, 4.8628) -> (13.2549, 4.6028) centre (13.2549, 4.9028) ccw
  arc A299 (10.7451, 4.6028) -> (11.0424, 4.8628) centre (10.7451, 4.9028) ccw
  line L229 (10.5, 4.6028) -> (10.7451, 4.6028)
  line L230 (13.2549, 4.6028) -> (13.5, 4.6028)
  arc A300 (12.9576, 4.8628) -> (12.5217, 5.8528) centre (11.025, 4.6028) ccw
  line L231 (11.4783, 5.8528) -> (12.5217, 5.8528)
  arc A301 (11.4783, 5.8528) -> (11.0424, 4.8628) centre (12.975, 4.6028) ccw
  arc A302 (9.9576, 4.8628) -> (10.2549, 4.6028) centre (10.2549, 4.9028) ccw
  arc A303 (7.7451, 4.6028) -> (8.0424, 4.8628) centre (7.7451, 4.9028) ccw
  line L232 (7.5, 4.6028) -> (7.7451, 4.6028)
  line L233 (10.2549, 4.6028) -> (10.5, 4.6028)
  arc A304 (9.9576, 4.8628) -> (9.5217, 5.8528) centre (8.025, 4.6028) ccw
  line L234 (8.4783, 5.8528) -> (9.5217, 5.8528)
  arc A305 (8.4783, 5.8528) -> (8.0424, 4.8628) centre (9.975, 4.6028) ccw
  arc A306 (6.9576, 4.8628) -> (7.2549, 4.6028) centre (7.2549, 4.9028) ccw
  arc A307 (4.7451, 4.6028) -> (5.0424, 4.8628) centre (4.7451, 4.9028) ccw
  line L235 (4.5, 4.6028) -> (4.7451, 4.6028)
  line L236 (7.2549, 4.6028) -> (7.5, 4.6028)
  arc A308 (6.9576, 4.8628) -> (6.5217, 5.8528) centre (5.025, 4.6028) ccw
  line L237 (5.4783, 5.8528) -> (6.5217, 5.8528)
  arc A309 (5.4783, 5.8528) -> (5.0424, 4.8628) centre (6.975, 4.6028) ccw
  arc A310 (3.9576, 4.8628) -> (4.2549, 4.6028) centre (4.2549, 4.9028) ccw
  arc A311 (1.7451, 4.6028) -> (2.0424, 4.8628) centre (1.7451, 4.9028) ccw
  line L238 (1.5, 4.6028) -> (1.7451, 4.6028)
  line L239 (4.2549, 4.6028) -> (4.5, 4.6028)
  arc A312 (3.9576, 4.8628) -> (3.5217, 5.8528) centre (2.025, 4.6028) ccw
  line L240 (2.4783, 5.8528) -> (3.5217, 5.8528)
  arc A313 (2.4783, 5.8528) -> (2.0424, 4.8628) centre (3.975, 4.6028) ccw
  arc A314 (0.9576, 4.8628) -> (1.2549, 4.6028) centre (1.2549, 4.9028) ccw
  arc A315 (-1.2549, 4.6028) -> (-0.9576, 4.8628) centre (-1.2549, 4.9028) ccw
  line L241 (-1.5, 4.6028) -> (-1.2549, 4.6028)
  line L242 (1.2549, 4.6028) -> (1.5, 4.6028)
  arc A316 (0.9576, 4.8628) -> (0.5217, 5.8528) centre (-0.975, 4.6028) ccw
  line L243 (-0.5217, 5.8528) -> (0.5217, 5.8528)